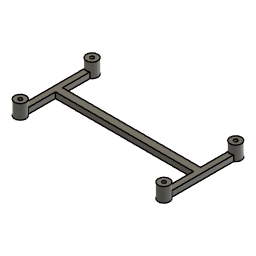
bracketReleGroupHouse (Autodesk Fusion 360 design; units mm, degrees)
Autodesk Fusion 360 part; units mm, degrees
sketch "Schizzo7" plane through (0, 0, 0) normal (0, 1, 0) x (1, 0, 0)
  line L0 (20, 10) -> (120.65, 10)
  line L1 (120.65, 10) -> (120.65, 60.3)
  line L2 (120.65, 60.3) -> (20, 60.3)
  line L3 (20, 60.3) -> (20, 10)
  circle A0 centre (120.65, 60.3) radius 4
  circle A1 centre (20, 60.3) radius 4
  circle A2 centre (20, 10) radius 4
  circle A3 centre (120.65, 10) radius 4
  line L4 (20, 60.3) -> (18, 60.3)
  line L5 (18, 60.3) -> (20, 60.3)
  line L6 (20, 60.3) -> (22, 60.3)
  line L7 (22, 60.3) -> (22, 10)
  line L8 (18, 60.3) -> (18, 10)
  line L9 (120.65, 60.3) -> (122.65, 60.3)
  line L10 (120.65, 60.3) -> (118.65, 60.3)
  line L11 (118.65, 60.3) -> (118.65, 10)
  line L12 (122.65, 60.3) -> (122.65, 10)
  line L13 (122.65, 10) -> (120.65, 10)
  line L14 (20, 35.15) -> (120.65, 35.15)
  line L15 (22, 35.15) -> (22, 37.65)
  line L16 (22, 35.15) -> (22, 32.65)
  line L17 (22, 37.65) -> (118.65, 37.65)
  line L18 (22, 32.65) -> (118.65, 32.65)
  dimension "d45" = 100.65
  dimension "d46" = 50.3
  dimension "d47" = 8
  dimension "d48" = 8
  dimension "d49" = 8
  dimension "d50" = 8
  dimension "d51" = 2
  dimension "d52" = 2
  dimension "d53" = 2.5
  dimension "d54" = 2.5
  constraint horizontal L0
  constraint vertical L1
  constraint horizontal L2
  constraint vertical L3
  constraint coincident L1.end L2.start
  constraint coincident L2.end L3.start
  constraint coincident L0.start L3.end
  constraint coincident L0.end L1.start
  constraint perpendicular L3 L4
  constraint coincident L2 L6.end
  constraint coincident L0 L7.end
  constraint perpendicular L0 L7
  constraint perpendicular L4 L8
  constraint perpendicular L1 L9
  constraint perpendicular L1 L10
  constraint coincident L0 L11.end
  constraint perpendicular L0 L11
  constraint perpendicular L9 L12
  constraint perpendicular L12 L13
  constraint midpoint L3 L14.start
  constraint midpoint L1 L14.end
  constraint midpoint L7 L15.start
  constraint perpendicular L14 L15
  constraint perpendicular L14 L16
  constraint coincident L11 L17.end
  constraint perpendicular L11 L17
  constraint coincident L11 L18.end
  constraint perpendicular L11 L18
  measures "d45" distance of L0.start L0.end
  measures "d46" distance of L0.start L2.end
  measures "d47" diameter of A0
  measures "d48" diameter of A1
  measures "d49" diameter of A2
  measures "d50" diameter of A3
  measures "d51" distance of L1.end L9.end
  measures "d52" distance of L1.end L10.end
  measures "d53" distance of L15.start L15.end
  measures "d54" distance of L15.start L16.end
extrude "Estrusione12" add sketch "Schizzo7" along normal blind 4 contours L3 A1 A2 L8 | L3 A2 L7 L14 L16 | L3 A1 L7 L14 L15 | L7 L11 L14 L16 L18 | L7 L11 L14 L15 L17 | L1 A3 L11 L14 | L1 A0 L11 L14 | L1 A0 A3 L12
extrude "Estrusione13" add sketch "Schizzo7" along normal blind 10 contours L0 L3 A2 L7 | L0 L3 A2 | L0 A2 L7 | L0 A3 L11 | L0 A3 L12 L13 | L3 A1 L4 L5 L8 | L2 L3 A1 L6 L7 | L2 A1 L4 L5 L6 L8 | L0 L1 A3 L11 | L2 A1 L7 | L1 A3 L12 L13 | L2 A0 L9 L10 L12 | L2 A0 L11 | L1 A0 L9 L12 | L1 L2 A0 L10 L11
hole "Foratura1" at (120.65, 10, -60.3) direction (0, -1, 0) diameter 2.5 depth 7 tip angle 118
hole "Foratura2" at (120.65, 10, -10) direction (0, -1, 0) diameter 2.5 depth 7 tip angle 118
hole "Foratura3" at (20, 10, -10) direction (0, -1, 0) diameter 2.5 depth 7 tip angle 118
hole "Foratura4" at (20, 10, -60.3) direction (0, -1, 0) diameter 2.5 depth 7 tip angle 118
